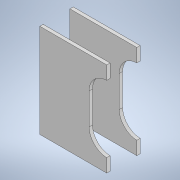
# Autodesk Inventor part: shooterCircularCurve
Saved by Autodesk Inventor 2022.2 (Build 262287000, 287)
## iProperties
Created: 2022-01-19
Part Number: shooterCircularCurve
Material: Generic
Document SubType Name: Modeling
Designer: robst
Density: 1 g/cm^3
Appearance: Default
Author: robst
Autodesk Inventor part; units mm, degrees
ref_plane "YZ Plane" through (0, 0, 0) normal (1, 0, 0) x (0, 1, 0)
ref_plane "XZ Plane" through (0, 0, 0) normal (0, 1, 0) x (-1, 0, 0)
ref_plane "Work Plane2" through (0, 0, 76.2) normal (0, 0, 1) x (1, 0, 0)
sketch "Sketch1" plane through (0, 0, 76.2) normal (0, 0, 1) x (1, 0, 0)
  line L0 (190.5, -190.5) -> (-190.5, -190.5)
  line L1 (-190.5, -190.5) -> (-190.5, 190.5)
  line L2 (-190.5, 190.5) -> (190.5, 190.5)
  line L3 (190.5, 190.5) -> (190.5, -190.5) construction
  line L4 (190.5, -190.5) -> (-190.5, 190.5) construction
  line L5 (-190.5, -190.5) -> (190.5, 190.5) construction
  line L6 (90.5263, 88.9) -> (90.5263, -88.9)
  arc A0 (190.5, 190.5) -> (90.5263, 88.9) centre (192.1395, 88.9) ccw
  arc A1 (90.5263, -88.9) -> (190.5, -190.5) centre (192.1395, -88.9) ccw
  line L7 (-190.5, 190.5) -> (190.5, 190.5)
  line L8 (190.5, 190.5) -> (190.5, 266.7)
  line L9 (190.5, 266.7) -> (-190.5, 266.7)
  line L10 (-190.5, 266.7) -> (-190.5, 190.5)
  line L11 (-190.5, -190.5) -> (190.5, -190.5)
  line L12 (190.5, -190.5) -> (190.5, -266.7)
  line L13 (190.5, -266.7) -> (-190.5, -266.7)
  line L14 (-190.5, -266.7) -> (-190.5, -190.5)
  point P0 (0, 0)
  dimension "d2" = 381
  dimension "d3" = 381
  dimension "d4" = 101.6
  dimension "d5" = 101.6
  dimension "d8" = 76.2
  dimension "d9" = 76.2
  constraints: 30 end point, 6 parallel, 4 point on circle, 3 horizontal, 3 perpendicular, 2 centre point, 2 midpoint, 2 tangent, 1 point on line, 1 vertical
  measures "d2" distance of L0.start L0.end
  measures "d3" distance of L0.end L1.end
  measures "d4" distance from line of L6.start L2
  measures "d5" distance from line of L6.end L0
  measures "d8" distance between parallel lines of L9 L2
  measures "d9" distance between parallel lines of L13 L0
extrude "Extrusion1" add sketch "Sketch1" along normal blind 19.05
mirror "Mirror1" about plane through (0, 0, 0) normal (0, 0, 1) of "Extrusion1"
equation "\"distanceBetweenPlates\" = 152.4"
equation "\"d1\" = 0.5 * distanceBetweenPlates"
body "Solid1"
